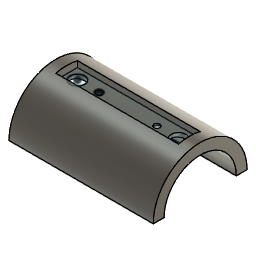
prototipo2_adaptador v1 (Autodesk Fusion 360 design; units mm, degrees)
Autodesk Fusion 360 part; units mm, degrees
sketch "Boceto1" plane through (0, 0, 0) normal (1, 0, 0) x (0, 1, 0)
  arc A0 (50, 0) -> (-50, 0) centre (0, 0) ccw
  line L0 (50, 0) -> (65, 0)
  line L1 (-50, 0) -> (-65, 0)
  arc A1 (65, 0) -> (-65, 0) centre (0, 0) ccw
  dimension "d3" = 100
  dimension "d27" = 15
  dimension "d28" = 15
  constraint horizontal A0.end A0.centre
  constraint horizontal L0
  constraint coincident A0.centre A1.centre
  constraint horizontal L1
  constraint concentric A0 A1
  constraint horizontal A0.start A0.centre
  measures "d3" diameter of A0
  measures "d27" distance of A0.start L0.end
  measures "d28" distance of A0.end L1.end
extrude "Extruir1" add sketch "Boceto1" along normal mid plane 200
sketch "Boceto4" plane through (106.6931, 0, 65) normal (0, 0, 1) x (1, 0, 0)
ref_plane "PlanoDeObra4" through (0, 0, 65) normal (0, 0, 1) x (0, -1, 0)
sketch "Boceto5" plane through (0, 0, 65) normal (0, 0, 1) x (1, 0, 0)
  line L0 (85, 15) -> (-85, 15)
  line L1 (-85, 15) -> (-85, -15)
  line L2 (-85, -15) -> (85, -15)
  line L3 (85, -15) -> (85, 15)
  line L4 (85, 15) -> (-85, -15) construction
  line L5 (-85, 15) -> (85, -15) construction
  dimension "d31" = 170
  dimension "d32" = 30
  constraint horizontal L0
  constraint perpendicular L0 L1
  constraint parallel L0 L2
  constraint parallel L1 L3
  constraint coincident L4 origin
  constraint coincident L5 origin
  measures "d31" distance of L1.end L2.end
  measures "d32" distance of L0.end L1.end
extrude "Extruir3" cut sketch "Boceto5" against normal blind 10
sketch "Boceto6" plane through (0, 0, 55) normal (0, 0, 1) x (-1, 0, 0)
  line L0 (-85, 15) -> (-85, -15)
  line L1 (-85, -15) -> (85, -15)
  line L2 (85, -15) -> (85, 15)
  line L3 (85, 15) -> (-85, 15)
  circle A0 centre (70, 0) radius 10
  circle A1 centre (40, 0) radius 5
  dimension "d35" = 20
  dimension "d36" = 10
  dimension "d37" = 15
  dimension "d38" = 15
  dimension "d39" = 30
  constraint horizontal A0.centre A1.centre
  measures "d35" diameter of A0
  measures "d36" diameter of A1
  measures "d37" distance of L2 A0.centre
  measures "d38" distance of L3 A0.centre
  measures "d39" distance of A0.centre A1.centre
hole "Agujero3" at (-40, 0, 55) direction (0, 0, -1) diameter 8.526 depth 2 tip angle 118
thread "Rosca2" "ISO Metric profile 10.0 M10x1.5 6H"
hole "Agujero4" at (-70, 0, 55) direction (0, 0, -1) diameter 20 end through all
ref_plane "PlanoDeObra5" through (0, 0, 60.9016) normal (1, 0, 0) x (0, -1, 0)
mirror "Simetría3" about plane through (0, 0, 60.9016) normal (1, 0, 0) of "Agujero3", "Agujero4"
